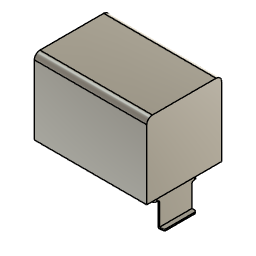
Poop Bucket (Autodesk Fusion 360 design; units mm, degrees)
Autodesk Fusion 360 part; units mm, degrees
note: some values were not read from the file. Set by a fixed rule: which face or edge a step refers to.
sketch "Sketch1" plane through (0, 0, 0) normal (0, 0, 1) x (1, 0, 0)
  line L0 (0, 0) -> (120, 0)
  line L1 (120, 0) -> (120, 80)
  line L2 (120, 80) -> (0, 80)
  line L3 (0, 80) -> (0, 0)
  dimension "d1" = 120
  dimension "d2" = 80
  constraint horizontal L0
  constraint vertical L1
  constraint horizontal L2
  constraint vertical L3
  constraint coincident L0.start L3.end
  measures "d1" distance of L0.start L0.end
  measures "d2" distance of L0.start L2.end
extrude "Extrude1" add sketch "Sketch1" along normal blind 80
fillet "Fillet1" radius 6 2 edges at (60, 80, 80) (60, 0, 80)
shell "Shell1" thickness 1 removed faces 1 at (0, 53.3333, 24.6667)
sketch "Sketch2" plane through (0, 0, 0) normal (0, 0, -1) x (1, 0, 0)
  line L0 (0, 0) -> (0, -80)
  line L1 (0, -80) -> (120, -80)
  line L2 (120, -80) -> (120, 0)
  line L3 (120, 0) -> (0, 0)
  line L4 (18, -18.25) -> (108, -18.25)
  line L5 (109.5, -19.75) -> (109.5, -60.25)
  line L6 (108, -61.75) -> (18, -61.75)
  line L7 (16.5, -60.25) -> (16.5, -19.75)
  arc A0 (18, -18.25) -> (16.5, -19.75) centre (18, -19.75) ccw
  arc A1 (16.5, -60.25) -> (18, -61.75) centre (18, -60.25) ccw
  arc A2 (109.5, -19.75) -> (108, -18.25) centre (108, -19.75) ccw
  arc A3 (108, -61.75) -> (109.5, -60.25) centre (108, -60.25) ccw
  point P0 (16.5, -18.25)
  point P1 (109.5, -18.25)
  point P2 (16.5, -61.75)
  dimension "d8" = 93
  dimension "d9" = 43.5
  dimension "d10" = 18.25
  dimension "d11" = 18.25
  dimension "d12" = 16.5
  dimension "d15" = 1.5
  dimension "d16" = 1.5
  constraint horizontal L4
  constraint vertical L5
  constraint horizontal L6
  constraint vertical L7
  constraint coincident P0 L4
  constraint coincident P0 L7
  constraint tangent L4 A0
  constraint tangent L7 A0
  constraint coincident P2 L6
  constraint coincident P2 L7
  constraint tangent L6 A1
  constraint tangent L7 A1
  constraint coincident P1 L4
  constraint coincident P1 L5
  constraint tangent L4 A2
  constraint tangent L5 A2
  constraint equal A1 A2
  constraint tangent L5 A3
  constraint tangent L6 A3
  constraint equal A1 A3
  measures "d8" distance of P0 P1
  measures "d9" distance of P0 P2
  measures "d10" distance of L3 L4
  measures "d11" distance of L1 L6
  measures "d12" distance of L0 L7
  measures "d15" radius of A0
  measures "d16" radius of A1
extrude "Extrude2" cut sketch "Sketch2" against normal up to surface (1 mm away) contours L4 L5 L6 L7 A0 A1 A2 A3
sketch "Sketch3" plane through (0, 0, 0) normal (0, 0, -1) x (1, 0, 0)
  line L0 (18, -18.25) -> (108, -18.25)
  arc A0 (109.5, -19.75) -> (108, -18.25) centre (108, -19.75) ccw
  line L1 (109.5, -19.75) -> (109.5, -60.25)
  arc A1 (108, -61.75) -> (109.5, -60.25) centre (108, -60.25) ccw
  line L2 (108, -61.75) -> (18, -61.75)
  arc A2 (16.5, -60.25) -> (18, -61.75) centre (18, -60.25) ccw
  line L3 (16.5, -60.25) -> (16.5, -19.75)
  arc A3 (18, -18.25) -> (16.5, -19.75) centre (18, -19.75) ccw
  line L4 (0, 0) -> (0, -80)
  line L5 (0, -80) -> (120, -80)
  line L6 (120, -80) -> (120, 0)
  line L7 (120, 0) -> (0, 0)
  arc A4 (111, -19.75) -> (108, -16.75) centre (108, -19.75) ccw
  line L8 (18, -16.75) -> (108, -16.75)
  arc A5 (18, -16.75) -> (15, -19.75) centre (18, -19.75) ccw
  line L9 (15, -60.25) -> (15, -19.75)
  arc A6 (15, -60.25) -> (18, -63.25) centre (18, -60.25) ccw
  line L10 (108, -63.25) -> (18, -63.25)
  arc A7 (108, -63.25) -> (111, -60.25) centre (108, -60.25) ccw
  line L11 (111, -19.75) -> (111, -60.25)
  dimension "d17" = -1.5
extrude "Extrude3" add sketch "Sketch3" along normal blind 11.5 contours A4 L8 A5 L9 A6 L10 A7 L11
sketch "Sketch4" plane through (0, 16.75, 0) normal (0, -1, 0) x (1, 0, 0)
  line L0 (108, 0) -> (18, 0)
  line L1 (18, 0) -> (18, -11.5)
  line L2 (18, -11.5) -> (108, -11.5)
  line L3 (108, -11.5) -> (108, 0)
  line L4 (15, 0) -> (15, -1.6) construction
  line L5 (15, -1.6) -> (29.14, -11.5)
  line L6 (15, 0) -> (15, -11.5)
  line L7 (29.14, -11.5) -> (15, -11.5)
  line L8 (15, -1.6) -> (15, -11.5)
  point P0 (15, -11.5)
  dimension "d20" = 1.6
  dimension "d21" = 14.14
  constraint vertical L4
  constraint coincident L2 L5.end
  constraint coincident L4.end L6
  constraint coincident P0 L6.end
  measures "d20" distance of L4.start L4.end
  measures "d21" distance of L5.end P0
extrude "Extrude4" cut sketch "Sketch4" against normal up to surface (46.5 mm away) contours L1 L2 L5 L7 | L1 L5 L6 L7 L8
fillet "Fillet2" radius 10 2 edges at (29.14, 17.5, -11.5) (29.14, 62.5, -11.5)
sketch "Sketch5" plane through (0, 0, -11.5) normal (0, 0, -1) x (1, 0, 0)
  line L0 (32.2927, -61.75) -> (32.2927, -63.25)
  line L1 (32.2927, -63.25) -> (108, -63.25)
  arc A0 (108, -63.25) -> (111, -60.25) centre (108, -60.25) ccw
  line L2 (111, -60.25) -> (111, -19.75)
  arc A1 (111, -19.75) -> (108, -16.75) centre (108, -19.75) ccw
  line L3 (108, -16.75) -> (32.2927, -16.75)
  line L4 (32.2927, -16.75) -> (32.2927, -18.25)
  line L5 (32.2927, -18.25) -> (108, -18.25)
  arc A2 (109.5, -19.75) -> (108, -18.25) centre (108, -19.75) ccw
  line L6 (109.5, -19.75) -> (109.5, -60.25)
  arc A3 (108, -61.75) -> (109.5, -60.25) centre (108, -60.25) ccw
  line L7 (108, -61.75) -> (32.2927, -61.75)
  line L8 (109.5, -22.75) -> (111, -22.75)
  line L9 (111, -22.75) -> (111, -57.25)
  line L10 (111, -57.25) -> (109.5, -57.25)
  line L11 (109.5, -57.25) -> (109.5, -22.75)
  dimension "d26" = 1.5
  dimension "d27" = 34.5
  dimension "d28" = 4.5
  dimension "d29" = 4.5
  constraint horizontal L8
  constraint vertical L9
  constraint horizontal L10
  constraint vertical L11
  constraint coincident L6 L8.start
  measures "d26" distance of L8.start L8.end
  measures "d27" distance of L8.start L10.end
  measures "d28" distance of L5 L8.start
  measures "d29" distance of L7 L10.end
extrude "Extrude5" add sketch "Sketch5" along normal blind 26.5 contours L2 L6 L8 L9 L10 L11
fillet "Fillet3" radius 2 2 edges at (110.25, 22.75, -11.5) (110.25, 57.25, -11.5)
sketch "Sketch6" plane through (111, 0, 0) normal (1, 0, 0) x (0, 1, 0)
  line L0 (60.25, 0) -> (19.75, 0)
  line L1 (19.75, 0) -> (19.75, -11.5)
  line L2 (19.75, -11.5) -> (20.75, -11.5)
  arc A0 (22.75, -13.5) -> (20.75, -11.5) centre (20.75, -13.5) ccw
  line L3 (22.75, -13.5) -> (22.75, -38)
  line L4 (22.75, -38) -> (57.25, -38)
  line L5 (57.25, -38) -> (57.25, -13.5)
  arc A1 (59.25, -11.5) -> (57.25, -13.5) centre (59.25, -13.5) ccw
  line L6 (59.25, -11.5) -> (60.25, -11.5)
  line L7 (60.25, -11.5) -> (60.25, 0)
  line L8 (22.75, -38) -> (57.25, -38)
  line L9 (57.25, -38) -> (57.25, -36.5)
  line L10 (57.25, -36.5) -> (22.75, -36.5)
  line L11 (22.75, -36.5) -> (22.75, -38)
  dimension "d34" = 34.5
  dimension "d35" = 1.5
  constraint horizontal L8
  constraint vertical L9
  constraint horizontal L10
  constraint vertical L11
  constraint coincident L3.end L4.start
  measures "d34" distance of L3.end L4.end
  measures "d35" distance of L3.end L10.end
extrude "Extrude6" add sketch "Sketch6" along normal blind 5 contours L3 L4 L5 L8 L9 L10 L11
fillet "Fillet4" radius 2 2 edges at (116, 57.25, -37.25) (116, 22.75, -37.25)
equation "d10 = d11"
equation "d28 = d29"
